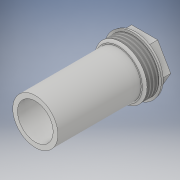
# Autodesk Inventor part: piston_corps
Saved by Autodesk Inventor 2019 (Build 230136000, 136)
## iProperties
Created: 2019-03-19
Part Number: piston_corps
Material: Générique
Document SubType Name: Modeling
Designer: theor
Density: 1 g/cm^3
Appearance: Par défaut
Author: theor
Autodesk Inventor part; units mm, degrees
ref_plane "YZ Plane" through (0, 0, 0) normal (1, 0, 0) x (0, 1, 0)
ref_plane "XZ Plane" through (0, 0, 0) normal (0, 1, 0) x (-1, 0, 0)
ref_plane "XY Plane" through (0, 0, 0) normal (0, 0, 1) x (1, 0, 0)
sketch "Esquisse1" plane through (0, 0, 0) normal (1, 0, 0) x (0, 1, 0)
  line L0 (0, 0) -> (0, -23.6667)
  line L1 (9.5, 0) -> (7.5, 0)
  line L2 (7.5, 0) -> (7.5, -43)
  line L3 (11, -35) -> (11, -41)
  line L4 (7.5, -43) -> (0, -43)
  line L5 (11, -46) -> (0, -46)
  line L6 (0, -43) -> (0, -46)
  line L7 (11, -46) -> (12, -41)
  line L8 (12, -41) -> (11, -41)
  line L9 (11, -35) -> (9.5, -35)
  line L10 (9.5, 0) -> (9.5, -35)
  dimension "d1" = 15
  dimension "d2" = 43
  dimension "d3" = 3
  dimension "d8" = 22
  dimension "d9" = 1
  dimension "d10" = 5
  dimension "d11" = 19
  dimension "d12" = 6
  constraints: 22 end point, 5 horizontal, 5 vertical, 1 collinear, 1 horizontal alignment, 1 vertical alignment
  measures "d1" diameter of L2 L0
  measures "d2" distance of L1.end L2.end
  measures "d3" distance of L4.end L5.end
  measures "d8" diameter of L3 L0
  measures "d9" distance of L7.end L3.end
  measures "d10" vertical distance of L5.start L7.end
  measures "d11" diameter of L10 L0
  measures "d12" distance between parallel lines of L8 L9
revolve "Révolution1" add sketch "Esquisse1" angle 360 about axis through (0, 0, 0) along (0, 0, -1)
chamfer "Chanfrein1" distance 1 angle 45 1 edges at (0, -7.5, -43)
sketch "Esquisse2" plane through (0, 0, -46) normal (0, 0, -1) x (-1, 0, 0)
  line L0 (5.4848, 9.5) -> (10.9697, 0)
  line L1 (10.9697, 0) -> (5.4848, -9.5)
  line L2 (5.4848, -9.5) -> (-5.4848, -9.5)
  line L3 (-5.4848, -9.5) -> (-10.9697, 0)
  line L4 (-10.9697, 0) -> (-5.4848, 9.5)
  line L5 (-5.4848, 9.5) -> (5.4848, 9.5)
  circle A0 centre (0, 0) radius 12 projected
  circle A1 centre (0, 0) radius 11 projected
  dimension "d13" = 19
  constraints: 12 end point, 1 coincident, 1 horizontal, 13 other
  measures "d13" distance between parallel lines of L2 L5
extrude "Extrusion1" cut sketch "Esquisse2" against normal blind 4 contours A0 | A1
thread "Filetage1" size "M22x1.5" class "6g" standard "ISO Metric profile" full length
chamfer "Chanfrein2" distance 1 angle 45 1 edges at (0, -11, -35)
